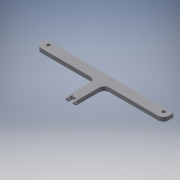
# Autodesk Inventor part: WebcamBase
Saved by Autodesk Inventor 2017 (Build 210142000, 142)
## iProperties
Created: 2015-05-12
Part Number: WebcamBase
Material: Generic
Document SubType Name: Modeling
Designer: Kurtis
Density: 1 g/cm^3
Appearance: Default
Author: Kurtis
Autodesk Inventor part; units mm, degrees
ref_plane "YZ Plane" through (0, 0, 0) normal (1, 0, 0) x (0, 1, 0)
ref_plane "XZ Plane" through (0, 0, 0) normal (0, 1, 0) x (-1, 0, 0)
ref_plane "XY Plane" through (0, 0, 0) normal (0, 0, 1) x (1, 0, 0)
sketch "Sketch1" plane through (0, 0, 0) normal (0, 0, 1) x (1, 0, 0)
  line L0 (254, 0) -> (254, 20)
  line L1 (254, 20) -> (0, 20)
  line L2 (0, 20) -> (0, 0)
  line L3 (0, 20) -> (0, 16) construction
  line L4 (0, 16) -> (8.5, 16) construction
  line L5 (8.5, 16) -> (11.75, 16) construction
  line L6 (11.75, 16) -> (11.75, 12.75) construction
  circle A0 centre (11.75, 12.75) radius 3.25
  line L7 (254, 20) -> (254, 16) construction
  line L8 (254, 16) -> (245.5, 16) construction
  line L9 (245.5, 16) -> (245.5, 12.75) construction
  line L10 (245.5, 12.75) -> (242.25, 12.75) construction
  circle A1 centre (242.25, 12.75) radius 3.25
  line L11 (0, 0) -> (254, 0)
  line L12 (127, 0) -> (127, -50) construction
  line L13 (122, -50) -> (132, -50)
  line L14 (132, -50) -> (132, -59)
  line L15 (122, -50) -> (122, -59)
  line L16 (132, -59) -> (136, -59)
  line L17 (122, -59) -> (118, -59)
  line L18 (118, -59) -> (118, 0)
  line L19 (136, -59) -> (136, 0)
  dimension "d1" = 20
  dimension "d2" = 4
  dimension "d3" = 8.5
  dimension "d4" = 3.25
  dimension "d5" = 3.25
  dimension "d6" = 4
  dimension "d7" = 8.5
  dimension "d8" = 3.25
  dimension "d9" = 3.25
  dimension "d14" = 242.25
  dimension "d40" = 50
  dimension "d41" = 10
  dimension "d42" = 5
  dimension "d43" = 0
  dimension "d44" = 9
  dimension "d45" = 9
  dimension "d46" = 4
  dimension "d47" = 4
  constraints: 40 end point, 7 perpendicular, 5 horizontal, 5 point on line, 4 vertical, 2 coincident, 1 horizontal alignment, 1 midpoint, 1 vertical alignment, 4 other
  measures "d1" distance of L0.start L0.end
  measures "d2" distance of L1.end L3.end
  measures "d3" distance of L3.end L4.end
  measures "d4" distance of L4.end L5.end
  measures "d5" distance of L5.end L6.end
  measures "d6" distance of L0.end L7.end
  measures "d7" distance of L7.end L8.end
  measures "d8" distance of L8.end L9.end
  measures "d9" distance of L9.end L10.end
  measures "d14" distance between parallel lines of L6 L0
  measures "d40" distance of L12.start L12.end
  measures "d41" distance of L13.start L13.end
  measures "d42" distance of L12.end L13.end
  measures "d43" distance from line of L12.end L13
  measures "d44" distance of L13.end L14.end
  measures "d45" distance of L13.start L15.end
  measures "d46" distance of L14.end L16.end
  measures "d47" distance of L15.end L17.end
extrude "Extrusion1" add sketch "Sketch1" along normal blind 8
fillet "Fillet2" radius 4 4 edges at (120, -59, 8) (120, -59, 0) (134, -59, 0) (134, -59, 8)
hole "Hole1" at (136, -55, 4) direction (-1, 0, 0) diameter 3 end through all
fillet "Fillet5" radius 10 4 edges at (0, 0, 4) (118, 0, 4) (136, 0, 4) (254, 0, 4)
fillet "Fillet6" radius 3 2 edges at (127, -50, 8) (127, -50, 0)
equation "\"d42\" = 0.5 * d41"
equation "\"d45\" = d44"
equation "\"d47\" = d46"
body "Solid1"
